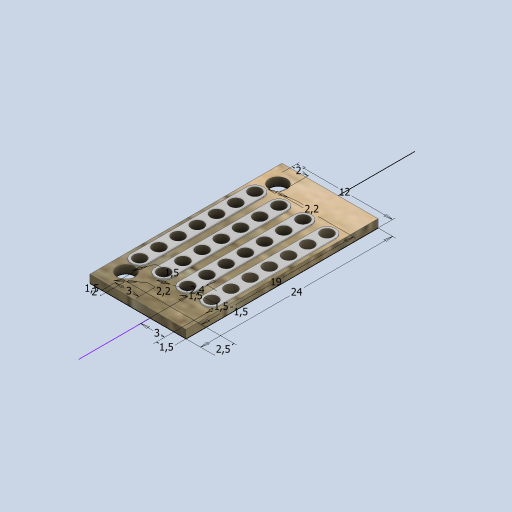
# Autodesk Inventor part: PDB
Saved by Autodesk Inventor 2023 (Build 270158000, 158)
## iProperties
Created: 2021-03-24
Part Number: PDB
Material: Generic
Document SubType Name: Modeling
Designer: JojoS
Density: 1 g/cm^3
Appearance: Default
Author: JojoS
Autodesk Inventor part; units mm, degrees
ref_plane "YZ Plane" through (0, 0, 0) normal (1, 0, 0) x (0, 1, 0)
ref_plane "XZ Plane" through (0, 0, 0) normal (0, 1, 0) x (-1, 0, 0)
sketch "Sketch1" plane through (0, 0, 0) normal (0, 1, 0) x (-1, 0, 0)
  line L0 (0, 0) -> (-12, 0)
  line L1 (-12, 0) -> (-12, -24)
  line L2 (-12, -24) -> (0, -24)
  line L3 (0, -24) -> (0, 0)
  circle A0 centre (-2, -2.5) radius 1.1
  circle A1 centre (-2, -21.5) radius 1.1
  circle A2 centre (-1.5, -4.7249) radius 0.75
  circle A3 centre (-10.5, -4.7249) radius 0.75
  circle A4 centre (-7.5, -4.7249) radius 0.75
  circle A5 centre (-4.5, -4.7249) radius 0.75
  circle A6 centre (-1.5, -7.1249) radius 0.75
  circle A7 centre (-4.5, -7.1249) radius 0.75
  circle A8 centre (-7.5, -7.1249) radius 0.75
  circle A9 centre (-10.5, -7.1249) radius 0.75
  circle A10 centre (-1.5, -9.5249) radius 0.75
  circle A11 centre (-4.5, -9.5249) radius 0.75
  circle A12 centre (-7.5, -9.5249) radius 0.75
  circle A13 centre (-10.5, -9.5249) radius 0.75
  circle A14 centre (-1.5, -11.9249) radius 0.75
  circle A15 centre (-4.5, -11.9249) radius 0.75
  circle A16 centre (-7.5, -11.9249) radius 0.75
  circle A17 centre (-10.5, -11.9249) radius 0.75
  circle A18 centre (-1.5, -14.3249) radius 0.75
  circle A19 centre (-4.5, -14.3249) radius 0.75
  circle A20 centre (-7.5, -14.3249) radius 0.75
  circle A21 centre (-10.5, -14.3249) radius 0.75
  circle A22 centre (-1.5, -16.7249) radius 0.75
  circle A23 centre (-4.5, -16.7249) radius 0.75
  circle A24 centre (-7.5, -16.7249) radius 0.75
  circle A25 centre (-10.5, -16.7249) radius 0.75
  circle A26 centre (-1.5, -19.1249) radius 0.75
  circle A27 centre (-4.5, -19.1249) radius 0.75
  circle A28 centre (-7.5, -19.1249) radius 0.75
  circle A29 centre (-10.5, -19.1249) radius 0.75
  line L4 (-7.5, 0) -> (-7.5, 8.9218)
  line L5 (-6, -24) -> (-6, -34.5946)
  circle A30 centre (-10, -2.5) radius 1.1
  circle A31 centre (-10, -21.5) radius 1.1
  dimension "d0" = 12
  dimension "d1" = 24
  dimension "d2" = 2.2
  dimension "d3" = 2.2
  dimension "d4" = 19
  dimension "d5" = 2.5
  dimension "d7" = 2
  dimension "d8" = 2
  dimension "d9" = 1.5
  dimension "d10" = 1.5
  dimension "d11" = 1.5
  dimension "d12" = 1.5
  dimension "d13" = 1.5
  dimension "d14" = 1.5
  dimension "d15" = 3
  dimension "d16" = 3
  dimension "d19" = 2.4
  constraints: 32 centre point, 12 end point, 3 vertical, 2 parallel, 2 symmetric about line, 1 horizontal, 1 midpoint, 1 perpendicular, 1 point on line, 50 other
  measures "d0" distance of L2.end L1.end
  measures "d1" distance of L1.end L0.end
  measures "d2" diameter of A0
  measures "d3" diameter of A1
  measures "d4" distance of A0.centre A1.centre
  measures "d5" distance from line of L0 A0.centre
  measures "d7" distance from line of L3 A0.centre
  measures "d8" distance from line of L3 A1.centre
  measures "d9" diameter of A2
  measures "d10" distance from line of L3 A2.centre
  measures "d11" diameter of A3
  measures "d12" diameter of A4
  measures "d13" diameter of A5
  measures "d14" distance from line of L1 A3.centre
  measures "d15" distance of A2.centre A5.centre
  measures "d16" distance of A3.centre A4.centre
  measures "d19" distance of A4.centre A8.centre
extrude "Extrusion1" add sketch "Sketch1" along normal blind 1 contours L3 L2 L1 L0 | A30 | A31
sketch "Sketch2" plane through (0, 1, 0) normal (0, 1, 0) x (1, 0, 0)
  line L0 (12, 24) -> (0, 24) projected
  line L1 (0, 24) -> (0, 0) projected
  line L2 (0, 0) -> (12, 0) projected
  line L3 (12, 0) -> (12, 24) projected
  circle A0 centre (10.5, 19.1249) radius 0.75 projected
  circle A1 centre (4.5, 19.1249) radius 0.75 projected
  circle A2 centre (10.5, 16.7249) radius 0.75 projected
  circle A3 centre (4.5, 16.7249) radius 0.75 projected
  circle A4 centre (10.5, 14.3249) radius 0.75 projected
  circle A5 centre (4.5, 14.3249) radius 0.75 projected
  circle A6 centre (10.5, 11.9249) radius 0.75 projected
  circle A7 centre (4.5, 11.9249) radius 0.75 projected
  circle A8 centre (10.5, 9.5249) radius 0.75 projected
  circle A9 centre (4.5, 9.5249) radius 0.75 projected
  circle A10 centre (10.5, 7.1249) radius 0.75 projected
  circle A11 centre (4.5, 7.1249) radius 0.75 projected
  circle A12 centre (1.5, 7.1249) radius 0.75 projected
  circle A13 centre (4.5, 4.7249) radius 0.75 projected
  circle A14 centre (7.5, 4.7249) radius 0.75 projected
  circle A15 centre (10.5, 4.7249) radius 0.75 projected
  circle A16 centre (1.5, 4.7249) radius 0.75 projected
  circle A17 centre (7.5, 7.1249) radius 0.75 projected
  circle A18 centre (1.5, 9.5249) radius 0.75 projected
  circle A19 centre (7.5, 9.5249) radius 0.75 projected
  circle A20 centre (1.5, 11.9249) radius 0.75 projected
  circle A21 centre (7.5, 11.9249) radius 0.75 projected
  circle A22 centre (1.5, 14.3249) radius 0.75 projected
  circle A23 centre (7.5, 14.3249) radius 0.75 projected
  circle A24 centre (1.5, 16.7249) radius 0.75 projected
  circle A25 centre (7.5, 16.7249) radius 0.75 projected
  circle A26 centre (1.5, 19.1249) radius 0.75 projected
  circle A27 centre (7.5, 19.1249) radius 0.75 projected
  circle A28 centre (1.5, 4.7249) radius 0.75 projected
  line L4 (1.5, 4.7249) -> (1.5, 19.1249) construction
  line L5 (2.55, 4.7249) -> (2.55, 19.1249)
  line L6 (0.45, 19.1249) -> (0.45, 4.7249)
  arc A29 (0.45, 4.7249) -> (2.55, 4.7249) centre (1.5, 4.7249) ccw
  arc A30 (2.55, 19.1249) -> (0.45, 19.1249) centre (1.5, 19.1249) ccw
  circle A31 centre (4.5, 4.7249) radius 0.75 projected
  circle A32 centre (4.5, 19.1249) radius 0.75 projected
  line L7 (4.5, 4.7249) -> (4.5, 19.1249) construction
  line L8 (5.55, 4.7249) -> (5.55, 19.1249)
  line L9 (3.45, 19.1249) -> (3.45, 4.7249)
  arc A33 (3.45, 4.7249) -> (5.55, 4.7249) centre (4.5, 4.7249) ccw
  arc A34 (5.55, 19.1249) -> (3.45, 19.1249) centre (4.5, 19.1249) ccw
  line L10 (7.5, 4.7249) -> (7.5, 19.1249) construction
  line L11 (8.55, 4.7249) -> (8.55, 19.1249)
  line L12 (6.45, 19.1249) -> (6.45, 4.7249)
  arc A35 (6.45, 4.7249) -> (8.55, 4.7249) centre (7.5, 4.7249) ccw
  arc A36 (8.55, 19.1249) -> (6.45, 19.1249) centre (7.5, 19.1249) ccw
  circle A37 centre (10.5, 4.7249) radius 0.75 projected
  line L13 (10.5, 4.7249) -> (10.5, 19.1249) construction
  line L14 (11.55, 4.7249) -> (11.55, 19.1249)
  line L15 (9.45, 19.1249) -> (9.45, 4.7249)
  arc A38 (9.45, 4.7249) -> (11.55, 4.7249) centre (10.5, 4.7249) ccw
  arc A39 (11.55, 19.1249) -> (9.45, 19.1249) centre (10.5, 19.1249) ccw
  point P0 (4.5, 11.9249)
  point P1 (7.5, 11.9249)
  point P2 (10.5, 11.9249)
  dimension "d26" = 2.1
  dimension "d27" = 2.1
  dimension "d28" = 2.1
  dimension "d29" = 2.1
  constraints: 32 end point, 16 point on circle, 16 tangent, 8 centre point, 7 parallel, 4 midpoint, 1 vertical
  measures "d26" diameter of A30
  measures "d27" diameter of A34
  measures "d28" diameter of A36
  measures "d29" diameter of A39
extrude "Extrusion2" add sketch "Sketch2" along normal blind 0.1 contours A29 L6 A30 L5 | A33 L9 A34 L8 | A35 L12 A36 L11 | A38 L15 A39 L14
ref_plane "Work Plane1" through (0, 0.5, 0) normal (0, 1, 0) x (1, 0, 0)
mirror "Mirror1" about plane through (0, 0.5, 0) normal (0, 1, 0) of "Extrusion2"
body "Solid1"
